Profile Joiner_v4 (Autodesk Fusion 360 design; units mm, degrees)
Autodesk Fusion 360 part; units mm, degrees
note: some values were not read from the file. Set by a fixed rule: which sketch regions a step uses.
sketch "Sketch1" plane through (0, 0, 0) normal (0, 0, 1) x (1, 0, 0)
  line L0 (1.8, 5.5) -> (3.4393, 5.5)
  line L1 (6.1, -2.8393) -> (3.4393, -5.5)
  line L2 (6.1, 2.8393) -> (6.1, -2.8393)
  line L3 (1.8, -5.5) -> (1.8, -3.2628)
  arc A0 (0.1778, -4.4022) -> (0.0013, -4.7917) centre (0.6071, -4.8314) ccw
  arc A1 (1.4586, 3.1214) -> (1.8, 3.2628) centre (1.6, 3.2628) ccw
  arc A2 (1.8, -3.2628) -> (1.4586, -3.1214) centre (1.6, -3.2628) ccw
  line L4 (3.4393, 5.5) -> (6.1, 2.8393)
  line L5 (3.4393, -5.5) -> (1.8, -5.5)
  arc A3 (0, 4.9) -> (0.1506, 4.4312) centre (0.6266, 4.8428) ccw
  line L6 (0.1506, 4.4312) -> (1.4586, 3.1214)
  line L7 (1.8, 3.2628) -> (1.8, 5.5)
  line L8 (1.4586, -3.1214) -> (0.1778, -4.4022)
  line L9 (0, 9.5) -> (0, 4.9)
  line L10 (0.0013, -4.7917) -> (0, -9.5)
  line L11 (-1.8, 5.5) -> (-3.4393, 5.5)
  line L12 (-6.1, -2.8393) -> (-3.4393, -5.5)
  line L13 (-6.1, 2.8393) -> (-6.1, -2.8393)
  line L14 (-1.8, -5.5) -> (-1.8, -3.2628)
  arc A4 (-0.1778, -4.4022) -> (-0.0013, -4.7917) centre (-0.607, -4.8314) cw
  arc A5 (-1.4586, 3.1214) -> (-1.8, 3.2628) centre (-1.6, 3.2628) cw
  arc A6 (-1.8, -3.2628) -> (-1.4586, -3.1214) centre (-1.6, -3.2628) cw
  line L15 (-3.4393, 5.5) -> (-6.1, 2.8393)
  line L16 (-3.4393, -5.5) -> (-1.8, -5.5)
  arc A7 (0, 4.9) -> (-0.1506, 4.4312) centre (-0.6266, 4.8428) cw
  line L17 (-0.1506, 4.4312) -> (-1.4586, 3.1214)
  line L18 (-1.8, 3.2628) -> (-1.8, 5.5)
  line L19 (-1.4586, -3.1214) -> (-0.1778, -4.4022)
  line L20 (0, 9.5) -> (0, 4.9)
  line L21 (-0.0013, -4.7917) -> (0, -9.5)
  line L22 (-0.1506, 4.4312) -> (0.1506, 4.4312)
  line L23 (-0.1778, -4.4022) -> (0.1778, -4.4022)
  line L24 (-0.05, 9.5) -> (-0.05, 4.9022)
  arc A8 (-0.05, 4.9022) -> (0.114, 4.3971) centre (0.6266, 4.8428) ccw
  line L25 (0.114, 4.3971) -> (1.423, 3.0863)
  arc A9 (1.423, 3.0863) -> (1.85, 3.2628) centre (1.6, 3.2628) ccw
  line L26 (1.85, 3.2628) -> (1.85, 5.45)
  line L27 (1.85, 5.45) -> (3.4186, 5.45)
  line L28 (3.4186, 5.45) -> (6.05, 2.8186)
  line L29 (6.05, 2.8186) -> (6.05, -2.8186)
  line L30 (6.05, -2.8186) -> (3.4186, -5.45)
  line L31 (3.4186, -5.45) -> (1.85, -5.45)
  line L32 (1.85, -5.45) -> (1.85, -3.2628)
  arc A10 (1.85, -3.2628) -> (1.4232, -3.0861) centre (1.6, -3.2628) ccw
  line L33 (1.4232, -3.0861) -> (0.1424, -4.3668)
  line L34 (-0.1506, 4.3312) -> (0.1506, 4.3312)
  line L35 (-0.1778, -4.3022) -> (0.1778, -4.3022)
  line L36 (0.2, 7.5) -> (-4.2678, 7.5)
  line L37 (-4.2678, 7.5) -> (-8.1, 3.6678)
  line L38 (-8.1, 3.6678) -> (-8.1, -3.6678)
  line L39 (-8.1, -3.6678) -> (-4.2678, -7.5)
  line L40 (-4.2678, -7.5) -> (0.2, -7.5)
  dimension "d1" = 2
  dimension "d2" = 0.05
  dimension "d3" = 0.1
  dimension "d4" = -0.1
  constraint horizontal L22
extrude "Extrude1" add sketch "Sketch1" along normal blind 10 contours L0 L1 L2 L3 A1 A2 L4 L5 L6 L7 L8 L11 L12 L13 L14 A5 A6 L15 L16 L17 L18 L19 L22 L23
